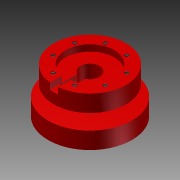
# Autodesk Inventor part: ToolHolderSpool
Saved by Autodesk Inventor 2012 SP1 (Build 160190100, 190)
## iProperties
Created: 2010-02-03
Part Number: ToolHolderSpool
Document SubType Name: Modeling
Designer: local-admin
Density: 2.71 g/cm^3
Material: Aluminum-6061
Mass: 83.3056 g
Surface Area: 138.876 cm^2
Volume: 30.7401 cm^3
Author: local-admin
Autodesk Inventor part; units mm, degrees
ref_plane "YZ Plane" through (0, 0, 0) normal (1, 0, 0) x (0, 1, 0)
ref_plane "XZ Plane" through (0, 0, 0) normal (0, 1, 0) x (-1, 0, 0)
ref_plane "XY Plane" through (0, 0, 0) normal (0, 0, 1) x (1, 0, 0)
sketch "Sketch1" plane through (0, 0, 0) normal (0, 0, 1) x (1, 0, 0)
  line L0 (0, -5.588) -> (0, 33.528) projected
  line L1 (-5.207, 0) -> (31.242, 0) projected
  line L2 (22.5044, 27.94) -> (22.5044, 17.4752)
  line L3 (22.5044, 17.4752) -> (12.5095, 17.4752)
  line L4 (12.5095, 17.4752) -> (12.5095, 10.4648)
  line L5 (12.5095, 10.4648) -> (26.035, 10.4648)
  line L6 (26.035, 10.4648) -> (26.035, 0)
  line L7 (22.5044, 27.94) -> (5.9563, 27.94)
  line L8 (26.035, 0) -> (24.8031, 0)
  line L9 (24.8031, 0) -> (24.8031, 2.2098)
  line L10 (24.8031, 2.2098) -> (22.1107, 2.2098)
  line L11 (22.1107, 2.2098) -> (22.1107, 0)
  line L12 (21, 0) -> (21, 8.89)
  line L13 (21, 8.89) -> (12.3952, 8.89)
  line L14 (12.3952, 8.89) -> (12.3952, 0)
  line L15 (10.5156, 0) -> (10.5156, 2.2098)
  line L16 (10.5156, 2.2098) -> (7.8486, 2.2098)
  line L17 (7.8486, 2.2098) -> (7.8486, 0)
  line L18 (4.0005, 1.524) -> (4.9149, 1.524)
  line L19 (4.9149, 1.524) -> (4.9149, 0)
  line L20 (4.0005, 1.524) -> (4.0005, 3.9243)
  line L21 (4.0005, 3.9243) -> (5.9563, 3.9243)
  line L22 (5.9563, 3.9243) -> (5.9563, 27.94)
  point P0 (0, 0)
  dimension "d1" = 22.5044
  dimension "d2" = 26.035
  dimension "d3" = 12.5095
  dimension "d7" = 10.4648
  dimension "d32" = 10.4648
  dimension "d33" = 27.94
  dimension "d36" = 21
  dimension "d37" = 4.9149
  dimension "d38" = 5.9563
  dimension "d39" = 4.0005
  dimension "d40" = 1.524
  dimension "d42" = 12.3952
  dimension "d43" = 8.89
  dimension "d86" = 24.8031
  dimension "d87" = 2.2098
  dimension "d88" = 22.1107
  dimension "d89" = 10.5156
  dimension "d90" = 7.8486
  dimension "d91" = 2.2098
  dimension "d105" = 24.0157
  constraints: 42 end point, 7 perpendicular, 5 vertical, 3 parallel, 2 horizontal, 9 other
  measures "d1" distance between parallel lines of L0 L2
  measures "d2" distance between parallel lines of L0 L6
  measures "d3" distance between parallel lines of L0 L4
  measures "d7" distance of the line from the sketch origin of L5
  measures "d32" distance of L2.start L2.end
  measures "d33" distance of the line from the sketch origin of L7
  measures "d36" distance between parallel lines of L0 L12
  measures "d37" distance between parallel lines of L0 L19
  measures "d38" distance between parallel lines of L0 L22
  measures "d39" distance between parallel lines of L0 L20
  measures "d40" distance of L18.end L19.end
  measures "d42" distance between parallel lines of L0 L14
  measures "d43" distance between parallel lines of L8 L13
  measures "d86" distance between parallel lines of L0 L9
  measures "d87" distance of the line from the sketch origin of L10
  measures "d88" distance between parallel lines of L0 L11
  measures "d89" distance between parallel lines of L0 L15
  measures "d90" distance between parallel lines of L0 L17
  measures "d91" distance of the line from the sketch origin of L16
  measures "d105" distance between parallel lines of L21 L7
revolve "Revolution1" add sketch "Sketch1" angle 360 about axis through (0, -10, 0) along (0, 1, 0) contours L19 L18 L20 L21 L22 L7 L2 L3 L4 L5 L6 L1 L9 L10 L11 L12 L13 L14 L15 L16 L17
sketch "Sketch4" plane through (0, 27.94, 0) normal (0, 1, 0) x (1, 0, 0)
  line L0 (0, 36.449) -> (0, -36.449) construction
  line L1 (0, 0) -> (6.697, 16.1679) construction
  circle A0 centre (0, 0) radius 22.5044 construction
  dimension "d100" = 17.5
  dimension "d102" = 22.5
  constraints: 2 end point, 1 coincident
  measures "d100" distance of L1.start L1.end
  measures "d102" angle of L1 L0
hole "Hole3" at (6.697, 27.94, -16.1679) direction (0, -1, 0) diameter 2.642 end up to face face through (18.9548, 17.4752, -1.7952) facing (0, -1, 0) thread size "6-32 UNC" class "2B" standard "ANSI Unified Screw Threads"
pattern_circular "Circular Pattern2" count 8 over 360 about axis through (0, 22.7076, 0) along (0, -1, 0) of "Hole3"
sketch "Sketch5" plane through (0, 27.94, 0) normal (0, 1, 0) x (1, 0, 0)
  circle A0 centre (0, 0) radius 22.5044 construction
  line L0 (0, 36.449) -> (0, -36.449) construction
  line L1 (0, -5.3876) -> (0, 0) construction
  circle A1 centre (0, 0) radius 5.9563 construction
  arc A2 (2.54, -14.898) -> (-2.54, -14.898) centre (0, 0) ccw
  line L2 (-2.54, -14.898) -> (-2.54, -22.3606)
  line L3 (2.54, -14.898) -> (2.54, -22.3606)
  arc A3 (-2.54, -22.3606) -> (2.54, -22.3606) centre (0, 0) ccw
  dimension "d57" = 0
  dimension "d106" = 30.226
  dimension "d107" = 2.54
  constraints: 6 end point, 4 point on circle, 2 centre point, 2 coincident, 2 symmetric about line, 1 vertical, 2 other
  measures "d57" distance between parallel lines of L1 L0
  measures "d106" diameter of A2
  measures "d107" distance between parallel lines of L0 L3
extrude "Extrusion1" cut sketch "Sketch5" against normal blind 3.9624
sketch "Sketch7" plane through (0, 23.9776, 0) normal (0, 1, 0) x (1, 0, 0)
  line L0 (-2.54, -14.898) -> (-2.54, -22.3606) construction
  line L1 (2.54, -22.3606) -> (2.54, -14.898) construction
  circle A0 centre (0, 0) radius 5.9563 construction
  line L2 (-2.54, -14.898) -> (-2.54, -5.3876)
  line L3 (2.54, -14.898) -> (2.54, -5.3876)
  arc A1 (-2.54, -14.898) -> (2.54, -14.898) centre (0, -14.898) ccw
  arc A2 (-2.54, -5.3876) -> (2.54, -5.3876) centre (0, 0) ccw
  constraints: 6 point on circle, 4 end point, 2 centre point, 2 parallel, 2 tangent, 1 concentric
extrude "Extrusion2" cut sketch "Sketch7" against normal up to surface (13.5128 mm away)
sketch "Sketch12" plane through (0, 10.4648, 0) normal (0, 1, 0) x (1, 0, 0)
  circle A0 centre (-11.79, -13.2405) radius 1.5875
  line L0 (-13.3775, -14.828) -> (-10.3336, -14.828) construction
  line L1 (-13.3775, -14.828) -> (-13.3775, -14.8349) construction
  line L2 (-31.6622, 12.5095) -> (42.5897, 12.5095) construction
  circle A1 centre (0, 0) radius 26.035 projected
  circle A2 centre (0, 0) radius 10.5156 projected
  dimension "d93" = 3.175
  dimension "d99" = 27.3375
  dimension "d103" = 12.5095
  dimension "d104" = 13.3775
  constraints: 6 end point, 2 tangent, 1 centre point, 1 horizontal, 1 parallel, 1 perpendicular
  measures "d93" diameter of A0
  measures "d99" distance between parallel lines of L0 L2
  measures "d103" distance from line of A2.centre L2
  measures "d104" horizontal distance of L1.end A1.centre
extrude "Extrusion4" cut sketch "Sketch12" against normal blind 15 contours A0
equation "\"d87\" = d91"
body "Solid1"
